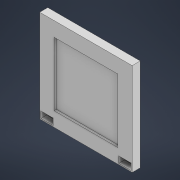
# Autodesk Inventor part: Circle_TestFit_V1
Saved by Autodesk Inventor 2022 (Build 260153000, 153)
## iProperties
Created: 2023-05-10
Part Number: Circle_TestFit_V1
Material: Generic
Document SubType Name: Modeling
Designer: Karl Spiteri
Density: 1 g/cm^3
Appearance: Default
Author: Karl Spiteri
Autodesk Inventor part; units mm, degrees
ref_plane "YZ Plane" through (0, 0, 0) normal (1, 0, 0) x (0, 1, 0)
ref_plane "XZ Plane" through (0, 0, 0) normal (0, 1, 0) x (-1, 0, 0)
ref_plane "XY Plane" through (0, 0, 0) normal (0, 0, 1) x (1, 0, 0)
sketch "Sketch1" plane through (0, 0, 0) normal (0, 0, 1) x (1, 0, 0)
  line L0 (0, 0) -> (-80, 0)
  line L1 (-80, 0) -> (-80, 80)
  line L2 (-80, 80) -> (0, 80)
  line L3 (0, 80) -> (0, 0)
  dimension "d4" = 80
  dimension "d5" = 80
  constraints: 8 end point, 2 parallel, 1 horizontal, 1 perpendicular
  measures "d4" distance of L1.end L2.end
  measures "d5" distance of L0.end L1.end
extrude "Extrusion2" add sketch "Sketch1" along normal blind 7
sketch "Sketch2" plane through (0, 0, 7) normal (0, 0, 1) x (1, 0, 0)
  line L0 (-12.5, 12.5) -> (-67.5, 12.5)
  line L1 (-67.5, 12.5) -> (-67.5, 67.5)
  line L2 (-67.5, 67.5) -> (-12.5, 67.5)
  line L3 (-12.5, 67.5) -> (-12.5, 12.5)
  point P0 (0, 0)
  dimension "d8" = 55
  dimension "d9" = 55
  constraints: 8 end point, 2 parallel, 1 horizontal, 1 perpendicular
  measures "d8" distance of L1.end L2.end
  measures "d9" distance of L0.end L1.end
extrude "Extrusion3" cut sketch "Sketch2" against normal blind 2
sketch "Sketch3" plane through (0, 0, 7) normal (0, 0, 1) x (1, 0, 0)
  line L0 (-1, 1) -> (-11.6, 1)
  line L1 (-11.6, 1) -> (-11.6, 6.6)
  line L2 (-11.6, 6.6) -> (-1, 6.6)
  line L3 (-1, 6.6) -> (-1, 1)
  line L4 (-79, 1) -> (-68.4, 1)
  line L5 (-68.4, 1) -> (-68.4, 6.6)
  line L6 (-68.4, 6.6) -> (-79, 6.6)
  line L7 (-79, 6.6) -> (-79, 1)
  point P0 (0, 0)
  dimension "d18" = 10.6
  dimension "d19" = 5.6
  dimension "d20" = 10.6
  dimension "d21" = 5.6
  constraints: 16 end point, 4 parallel, 2 horizontal, 2 perpendicular
  measures "d18" distance of L1.end L2.end
  measures "d19" distance of L0.end L1.end
  measures "d20" distance of L6.end L5.end
  measures "d21" distance of L5.end L4.end
extrude "Extrusion5" cut sketch "Sketch3" against normal blind 5
body "Solid2"
